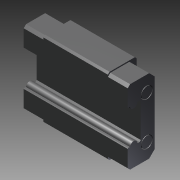
# Autodesk Inventor part: LU15ALW/O_slider_1
Saved by Autodesk Inventor 2011 SP1 (Build 150282100, 282)
## iProperties
Created: 2015-07-20
Part Number: LU15ALW/O_slider_1
Catalog Web Link: www.cadenas.de
Description: lu_slider_1-lu_slider_1
Vendor: NSK_RB
Document SubType Name: Modeling
Designer: PARTuser1
Manufacturer: NSK_RB
Mass: 12.5539 g
Surface Area: 53.0906 cm^2
Volume: 12.5539 cm^3
Density: 1 g/cm^3
Category: PARTsolutions
Company: NSK_RB
Title: LU15AL
Author: Cadenas PARTsolutions
Comments: lu_slider_1
PSOL_IDENT_0: {$CADENAS_DATA\23d-libs\nsk_rb\nsk_linear_products\nsk_linear_guides\standard_series\lu_series\lu_al
PSOL_IDENT_1: _series\parts\lu_slider.prj},174 {VTYP=3D},{NB=LU15ALW/O_slider_1},{LINA=LU15AL},{NN=lu_slider_1},{D
PSOL_IDENT_2: ATE=18.06.2013 02:53:32},{GEOMDATE=26.08.2009 00:00:00},{VERSION=},{LINEID=740},{LINESUBID=-1},{WBVA
PSOL_IDENT_3: R=SS}  {NB=LU15ALW/O_slider_1},{LINA=LU15AL},{KT=DUMMY},{PN=LU15ALW/O_slider_1},{MN=LU15AL},{ALG=LU1
PSOL_IDENT_4: 5AL},{SS=W/O},{SSALG='W/O','Without Side seal'},{MNA=AL},{S=15},{H=16.0},{E=4.0},{W2=8.5},{W=32},{L=
PSOL_IDENT_5: 43.600},{B=25},{J=20},{M=3.0},{TL=4.0},{B1=3.5},{L1=27.000},{J1=3.40},{K=12.0},{W1=15},{H1=9.5},{F=4
PSOL_IDENT_6: 0},{D=3.500},{DD=6.000},{HH=4.500},{B3=7.5},{DT=3.5},{DDT=6},{HHT=4.5},{LX=0.0000},{AD1=4.5000},{AD2=
PSOL_IDENT_7: 5.0000},{AX1=7.0000},{AX2=4.0000},{A1=7.000},{A2=4.0000}
SUPPLIER: NSK_RB
ARTICLENO: LU15ALW/O_slider_1
BOMINFO: LU15AL
CREATOR: CADENAS GmbH
Autodesk Inventor part; units mm, degrees
sketch "Sketch_31" plane through (0, 0, 0) normal (1, 0, 0) x (0, 0, -1)
  line L0 (-15.5, 9) -> (-15.5, 1)
  line L1 (-15.5, 1) -> (-14.5, 0)
  line L2 (-14.5, 0) -> (14.4999, 0)
  line L3 (14.4999, 0) -> (15.5, 1)
  line L4 (15.5, 1) -> (15.5, 9)
  line L5 (15.5, 9) -> (13.15, 11.35)
  line L6 (13.15, 11.35) -> (-13.15, 11.35)
  line L7 (-13.15, 11.35) -> (-15.5, 9)
  constraints: 16 end point
extrude "Extrusion1" add sketch "Sketch_31" along normal blind 43.6
sketch "Sketch_32" plane through (8.3, 0, 0) normal (1, 0, 0) x (0, 0, -1)
  line L0 (-16, 0.7) -> (-15.3, 0)
  line L1 (-15.3, 0) -> (15.3, 0)
  line L2 (15.3, 0) -> (16, 0.7)
  line L3 (16, 0.7) -> (16, 11.3)
  line L4 (16, 11.3) -> (15.3, 12)
  line L5 (15.3, 12) -> (8, 12)
  line L6 (8, 12) -> (7.6, 11.6)
  line L7 (7.6, 11.6) -> (-7.6, 11.6)
  line L8 (-7.6, 11.6) -> (-7.9999, 12)
  line L9 (-7.9999, 12) -> (-15.2999, 12)
  line L10 (-15.2999, 12) -> (-16, 11.3)
  line L11 (-16, 11.3) -> (-16, 0.7)
  constraints: 24 end point
extrude "Extrusion2" add sketch "Sketch_32" along normal blind 27
sketch "Sketch_33" plane through (0, 0, 0) normal (1, 0, 0) x (0, 0, -1)
  line L0 (-7.5, 5) -> (-7.5, 4.1225)
  arc A0 (-7.25, 0.9321) -> (-7.5, 4.1225) centre (-7.5, 2.5175) ccw
  line L1 (-7.25, 0.9321) -> (-7.25, 0.25)
  line L2 (-7.25, 0.25) -> (-7.5, 0)
  line L3 (-7.5, 0) -> (-7.5, -3.5)
  line L4 (-7.5, -3.5) -> (-7, -4)
  line L5 (-7, -4) -> (6.9999, -4)
  line L6 (6.9999, -4) -> (7.5, -3.5)
  line L7 (7.5, -3.5) -> (7.5, 0)
  line L8 (7.5, 0) -> (7.25, 0.25)
  line L9 (7.25, 0.25) -> (7.25, 0.9321)
  arc A1 (7.5, 4.1225) -> (7.25, 0.9321) centre (7.5, 2.5175) ccw
  line L10 (7.5, 4.1225) -> (7.5, 5)
  line L11 (7.5, 5) -> (7, 5.5)
  line L12 (7, 5.5) -> (-7, 5.5)
  line L13 (-7, 5.5) -> (-7.5, 5)
  constraints: 28 end point, 4 point on circle, 2 centre point
extrude "Extrusion3" cut sketch "Sketch_33" along normal blind 43.6
sketch "Sketch4" plane through (8.3, 12, 15.2999) normal (0, 1, 0) x (1, 0, 0)
  point P0 (3.4, 2.7999)
hole "Hole1" at (11.7, 12, 12.5) direction (0, -1, 0) diameter 2.459 depth 5.2 tip angle 120 countersink diameter 3 countersink angle 90 thread size "M3x0.5" class "6H" standard "ISO Metric profile"
pattern_linear "Rectangular Pattern1" count 2 spacing 20 along (1, 0, 0) count 2 spacing 25 along (0, 0, -1) of "Hole1"
sketch "Sketch_56" plane through (0, 0, 0) normal (1, 0, 0) x (0, 1, 0)
  circle A0 centre (8, 9) radius 2.49
  circle A1 centre (8, 9) radius 2.25
  constraints: 2 centre point
extrude "Extrusion4" cut sketch "Sketch_56" along normal blind 2.18
sketch "Sketch_61" plane through (0, 0, 0) normal (1, 0, 0) x (0, 1, 0)
  circle A0 centre (8, -9) radius 2.49
  circle A1 centre (8, -9) radius 2.25
  constraints: 2 centre point
extrude "Extrusion5" cut sketch "Sketch_61" along normal blind 2.18
sketch "Sketch_60" plane through (43.6, 0, 0) normal (1, 0, 0) x (0, 0, -1)
  circle A0 centre (-9, 8) radius 2.49
  circle A1 centre (-9, 8) radius 2.25
  constraints: 2 centre point
extrude "Extrusion6" cut sketch "Sketch_60" against normal blind 2.18
sketch "Sketch_63" plane through (43.6, 0, 0) normal (1, 0, 0) x (0, 0, -1)
  circle A0 centre (9, 8) radius 2.49
  circle A1 centre (9, 8) radius 2.25
  constraints: 2 centre point
extrude "Extrusion7" cut sketch "Sketch_63" against normal blind 2.18
ref_plane "slider_XY" through (0, 0, 0) normal (1, 0, 0) x (0, 0, -1)
ref_plane "slider_YZ" through (0, 0, 0) normal (0, 0, -1) x (0, 1, 0)
ref_plane "slider_ZX" through (0, 0, 0) normal (0, 1, 0) x (1, 0, 0)
body "Solid1"
